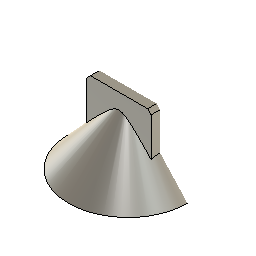
Mower key umbrella (Autodesk Fusion 360 design; units mm, degrees)
Autodesk Fusion 360 part; units mm, degrees
sketch "Sketch1" plane through (0, 0, 0) normal (0, 1, 0) x (1, 0, 0)
  line L0 (-12.1, -17.5) -> (-13.8, 0)
  line L1 (-12.1, -17.5) -> (-11.5171, -23.5)
  line L2 (-13.8, 0) -> (0, 0)
  line L3 (0, 0) -> (0, -23.5) construction
  line L4 (-12.1, -17.5) -> (0, -17.5) construction
  line L5 (-11.5171, -23.5) -> (0, -23.5)
  line L6 (0, 0) -> (0, -23.5) construction
  line L7 (13.8, 0) -> (0, 0)
  line L8 (12.1, -17.5) -> (13.8, 0)
  line L9 (11.5171, -23.5) -> (0, -23.5)
  line L10 (12.1, -17.5) -> (11.5171, -23.5)
  line L11 (0, -29.5) -> (33.5, 4) construction
  line L12 (33.5, 4) -> (33.5, 7.6922)
  line L13 (0, -29.5) -> (14.1, -29.5)
  line L14 (14.1, -29.5) -> (14.1, -15.4)
  line L15 (0, -29.5) -> (-14.1, -29.5)
  line L16 (-14.1, -29.5) -> (-14.1, -15.4)
  line L17 (14.1, -15.4) -> (-14.1, -15.4)
  line L18 (33.5, 4) -> (28.0093, 4)
  line L19 (28.0093, 4) -> (0, 4)
  line L20 (0, 4) -> (0, -29.5)
  line L21 (3, -29.5) -> (33.5, 4)
  line L22 (13.8, 0) -> (16.1094, 4)
  line L23 (-13.8, 0) -> (-16.1094, 4)
  line L24 (-28.0093, 4) -> (0, 4)
  dimension "d1" = 17.5
  dimension "d4" = 6
  dimension "d7" = 27.6
  dimension "d8" = 24.2
  dimension "d13" = 135
  dimension "d14" = 2
  dimension "d15" = 6
  dimension "d16" = 4
  dimension "d22" = 3
  dimension "d26" = 60
  constraint parallel L0 L1
  constraint coincident L2.end L3.start
  constraint horizontal L2
  constraint coincident L3 L4.end
  constraint perpendicular L3 L4
  constraint horizontal L4
  constraint perpendicular L3 L5
  constraint symmetric L0.start L3 L8.start
  constraint symmetric L0.end L3 L7.start
  constraint symmetric L1.end L3 L9.start
  constraint symmetric L2.end L3 L6.start
  constraint symmetric L5.end L3 L6.end
  constraint coincident L3 L11.start
  constraint vertical L12
  constraint horizontal L13
  constraint coincident L11 L14.end
  constraint perpendicular L13 L14
  constraint symmetric L6 L11.start L13.start
  constraint symmetric L6 L13.end L15.end
  constraint symmetric L6 L14.end L16.end
  constraint perpendicular L12 L18
  constraint perpendicular L3 L19
  constraint perpendicular L13 L20
  constraint coincident L13 L21.start
  constraint coincident L19 L22.end
  constraint symmetric L7.start L20 L0.end
  constraint symmetric L18.end L20 L24.start
  constraint symmetric L19.end L20 L24.end
  constraint symmetric L20 L22.end L23.end
  measures "d1" vertical distance of L0.start L0.end
  measures "d4" vertical distance of L0.start L1.end
  measures "d7" distance of L0.end L7.start
  measures "d8" distance of L0.start L8.start
  measures "d13" angle of L11 L12
  measures "d14" distance of L8.start L14
  measures "d15" distance of L1.end L15
  measures "d16" vertical distance of L7.start L11.end
  measures "d22" distance of L11.start L21.start
  measures "d26" angle of L19 L22
extrude "Extrude1" add sketch "Sketch1" along normal mid plane 6.1 contours L0 L1 L5 L17 L20 | L0 L2 L17 L20 | L2 L20 L23 L24 | L7 L8 L17 L20 | L8 L9 L10 L17 L20 L21 | L7 L19 L20 L22 | L9 L10 L21 makes body 1
fillet "Fillet1" radius 0.4 2 edges at (11.5171, 0, 23.5) (-11.5171, 0, 23.5) on bodies 1
revolve "Revolve1" add sketch "Sketch1" angle 360 about axis through (0, 0, -4) along (0, 0, 1) separate body contours L7 L8 L17 L20 | L8 L9 L10 L17 L20 L21 | L9 L13 L20 L21 | L7 L19 L20 L22 | L8 L10 L14 L17 L21 | L8 L14 L17 L18 L19 L21 L22 makes body 2
sketch "Sketch3" plane through (0, 0, -4) normal (0, 0, -1) x (1, 0, 0)
  circle A0 centre (0, 0) radius 33.5
  line L0 (-16.1094, 3.05) -> (-16.1094, -3.05) construction
  line L1 (-16.1094, -3.05) -> (16.1094, -3.05) construction
  line L2 (16.1094, -3.05) -> (16.1094, 3.05) construction
  line L3 (16.1094, 3.05) -> (-16.1094, 3.05) construction
  line L4 (18.1094, 5.05) -> (-18.1094, 5.05)
  line L5 (-18.1094, 5.05) -> (-18.1094, -5.05)
  line L6 (-18.1094, -5.05) -> (18.1094, -5.05)
  line L7 (18.1094, -5.05) -> (18.1094, 5.05)
  dimension "d27" = 2
extrude "Extrude3" add sketch "Sketch3" against normal blind 40 contours L4 L5 L6 L7 bodies 2
combine "Combine1" operation cut target body 2 tool bodies 1
chamfer "Chamfer1" distance 2 angle 45 2 edges at (18.1094, 0, 36) (-18.1094, 0, 36) on bodies 2
sketch "Sketch4" plane through (0, 0, 0) normal (0, 1, 0) x (1, 0, 0)
  line L0 (18.1094, -12.9044) -> (33.5, 4)
  line L1 (-33.5, 4) -> (-18.1094, -12.9044)
  line L2 (33.5, 4) -> (27.5, 4)
  line L3 (27.5, 4) -> (23.8582, 0)
  line L4 (23.8582, 0) -> (0, 0)
  line L5 (0, 0) -> (0, 4)
  line L6 (0, 4) -> (27.5, 4)
  point P0 (-33.5, 4)
  point P1 (33.5, 4)
  dimension "d29" = 6
  constraint coincident P1 L0.end
  constraint horizontal L2
  constraint parallel L0 L3
  constraint coincident L4.end L5.start
  constraint horizontal L4
  constraint perpendicular L2 L5
  constraint perpendicular L5 L6
  measures "d29" distance of P1 L2.end
revolve "Revolve2" cut sketch "Sketch4" angle 360 about axis through (0, 0, 1.75) along (0, 0, 1) bodies 2
named bodies: "Hole for key", "Key Cover"
